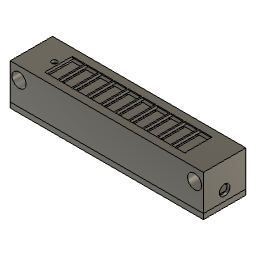
USB Power Distribution (Autodesk Fusion 360 design; units mm, degrees)
Autodesk Fusion 360 part; units mm, degrees
note: some values were not read from the file. Set by a fixed rule: which sketch regions a step uses.
sketch "Sketch1" plane through (0, 0, 0) normal (0, 0, 1) x (1, 0, 0) in component "USB PCB"
  line L0 (2, 0) -> (87.5, 0)
  line L1 (89.5, 2) -> (89.5, 16)
  line L2 (87.5, 18) -> (2, 18)
  line L3 (0, 16) -> (0, 2)
  circle A0 centre (2.7, 2.5) radius 1.75
  circle A1 centre (2.5, 15.5) radius 1.75
  circle A2 centre (87, 2.5) radius 1.75
  circle A3 centre (87, 15.5) radius 1.75
  arc A4 (2, 18) -> (0, 16) centre (2, 16) ccw
  arc A5 (89.5, 16) -> (87.5, 18) centre (87.5, 16) ccw
  arc A6 (87.5, 0) -> (89.5, 2) centre (87.5, 2) ccw
  arc A7 (0, 2) -> (2, 0) centre (2, 2) ccw
  line L4 (12.6, 1.25) -> (5.4, 1.25)
  line L5 (5.4, 1.25) -> (5.4, 16.75)
  line L6 (5.4, 16.75) -> (12.6, 16.75)
  line L7 (12.6, 16.75) -> (12.6, 1.25)
  line L8 (12.6, 1.25) -> (5.4, 16.75) construction
  line L9 (5.4, 1.25) -> (12.6, 16.75) construction
  line L10 (13.4, 16.75) -> (20.6, 16.75)
  line L11 (13.4, 1.25) -> (13.4, 16.75)
  line L12 (20.6, 16.75) -> (20.6, 1.25)
  line L13 (20.6, 1.25) -> (13.4, 1.25)
  line L14 (21.4, 16.75) -> (28.6, 16.75)
  line L15 (21.4, 1.25) -> (21.4, 16.75)
  line L16 (28.6, 16.75) -> (28.6, 1.25)
  line L17 (28.6, 1.25) -> (21.4, 1.25)
  line L18 (29.4, 16.75) -> (36.6, 16.75)
  line L19 (29.4, 1.25) -> (29.4, 16.75)
  line L20 (36.6, 16.75) -> (36.6, 1.25)
  line L21 (36.6, 1.25) -> (29.4, 1.25)
  line L22 (37.4, 16.75) -> (44.6, 16.75)
  line L23 (37.4, 1.25) -> (37.4, 16.75)
  line L24 (44.6, 16.75) -> (44.6, 1.25)
  line L25 (44.6, 1.25) -> (37.4, 1.25)
  line L26 (45.4, 16.75) -> (52.6, 16.75)
  line L27 (45.4, 1.25) -> (45.4, 16.75)
  line L28 (52.6, 16.75) -> (52.6, 1.25)
  line L29 (52.6, 1.25) -> (45.4, 1.25)
  line L30 (53.4, 16.75) -> (60.6, 16.75)
  line L31 (53.4, 1.25) -> (53.4, 16.75)
  line L32 (60.6, 16.75) -> (60.6, 1.25)
  line L33 (60.6, 1.25) -> (53.4, 1.25)
  line L34 (61.4, 16.75) -> (68.6, 16.75)
  line L35 (61.4, 1.25) -> (61.4, 16.75)
  line L36 (68.6, 16.75) -> (68.6, 1.25)
  line L37 (68.6, 1.25) -> (61.4, 1.25)
  line L38 (69.4, 16.75) -> (76.6, 16.75)
  line L39 (69.4, 1.25) -> (69.4, 16.75)
  line L40 (76.6, 16.75) -> (76.6, 1.25)
  line L41 (76.6, 1.25) -> (69.4, 1.25)
  line L42 (77.4, 16.75) -> (84.6, 16.75)
  line L43 (77.4, 1.25) -> (77.4, 16.75)
  line L44 (84.6, 16.75) -> (84.6, 1.25)
  line L45 (84.6, 1.25) -> (77.4, 1.25)
  circle A8 centre (3, 9) radius 2
  point P0 (89.5, 18)
  point P1 (0, 18)
  point P2 (9, 9)
  dimension "d1" = 18
  dimension "d2" = 89.5
  dimension "d3" = 3.5
  dimension "d4" = 2.7
  dimension "d5" = 3.5
  dimension "d6" = 2.5
  dimension "d7" = 3.5
  dimension "d8" = 3.5
  dimension "d9" = 15.5
  dimension "d10" = 2.5
  dimension "d11" = 87
  dimension "d12" = 2.5
  dimension "d13" = 87
  dimension "d14" = 15.5
  dimension "d15" = 2
  dimension "d16" = 2
  dimension "d17" = 9
  dimension "d18" = 15.5
  dimension "d19" = 9
  dimension "d20" = 7.2
  dimension "d23" = 8
  dimension "d24" = 0
  dimension "d29" = 4
  dimension "d30" = 3
  constraint horizontal L0
  constraint vertical L1
  constraint horizontal L2
  constraint vertical L3
  constraint coincident P1 L2
  constraint coincident P1 L3
  constraint tangent L2 A4
  constraint tangent L3 A4
  constraint coincident P0 L1
  constraint coincident P0 L2
  constraint tangent L1 A5
  constraint tangent L2 A5
  constraint tangent L0 A6
  constraint tangent L1 A6
  constraint equal A5 A6
  constraint coincident origin L0
  constraint coincident origin L3
  constraint tangent L0 A7
  constraint tangent L3 A7
  constraint equal A5 A7
  constraint perpendicular L4 L5
  constraint parallel L4 L6
  constraint parallel L5 L7
  constraint horizontal L4
  constraint coincident L8 P2
  constraint coincident L9 P2
  measures "d1" distance of origin P1
  measures "d2" distance of P0 P1
  measures "d3" diameter of A0
  measures "d4" distance of L3 A0.centre
  measures "d5" diameter of A1
  measures "d6" distance of L3 A1.centre
  measures "d7" diameter of A2
  measures "d8" diameter of A3
  measures "d9" distance of L0 A1.centre
  measures "d10" distance of L0 A0.centre
  measures "d11" distance of L3 A2.centre
  measures "d12" distance of L0 A2.centre
  measures "d13" distance of L3 A3.centre
  measures "d14" distance of L0 A3.centre
  measures "d15" radius of A4
  measures "d16" radius of A5
  measures "d17" distance of L3 P2
  measures "d18" distance of L4.start L6.end
  measures "d19" distance of L0 P2
  measures "d20" distance of L5 L7
  measures "d29" diameter of A8
  measures "d30" distance of L3 A8.centre
extrude "Extrude3" add sketch "Sketch1" along normal blind 7.5 contours A8 makes body 1 in component "USB PCB"
extrude "Extrude1" add sketch "Sketch1" against normal blind 1.6 separate body contours L0 L1 L2 L3 A4 A5 A6 A7 | L4 L5 L6 L7 | L10 L11 L12 L13 | L14 L15 L16 L17 | L18 L19 L20 L21 | L22 L23 L24 L25 | L26 L27 L28 L29 | L30 L31 L32 L33 | L34 L35 L36 L37 | L38 L39 L40 L41 | L42 L43 L44 L45 | A8 makes body 2 in component "USB PCB"
extrude "Extrude2" add sketch "Sketch1" along normal blind 13 contours L4 L5 L6 L7 | L10 L11 L12 L13 | L14 L15 L16 L17 | L18 L19 L20 L21 | L22 L23 L24 L25 | L26 L27 L28 L29 | L30 L31 L32 L33 | L34 L35 L36 L37 | L38 L39 L40 L41 | L42 L43 L44 L45 bodies 2 in component "USB PCB"
fillet "Fillet1" radius 2 1 edges at (1.1353, 8.2768, 7.5) on bodies 1 in component "USB PCB"
sketch "Sketch1 (2)" plane through (0, 0, 0) normal (0, 0, 1) x (1, 0, 0) in component "Bottom"
  line L0 (-10, 21) -> (99.5, 21)
  line L1 (99.5, 21) -> (99.5, -3)
  line L2 (99.5, -3) -> (-10, -3)
  line L3 (-10, -3) -> (-10, 21)
  line L4 (0, 16) -> (0, 2)
  line L5 (89.5, 2) -> (89.5, 16)
  circle A0 centre (87, 15.5) radius 3.25
  circle A1 centre (87, 2.5) radius 3.25
  circle A2 centre (2.5, 15.5) radius 3.25
  circle A3 centre (2.7, 2.5) radius 3.25
  line L6 (97.7, 19.2) -> (97.7, -1.2)
  line L7 (97.7, -1.2) -> (-8.2, -1.2)
  line L8 (-8.2, -1.2) -> (-8.2, 19.2)
  line L9 (-8.2, 19.2) -> (97.7, 19.2)
  line L10 (96.1, 0.4) -> (-6.6, 0.4)
  line L11 (-6.6, 0.4) -> (-6.6, 17.6)
  line L12 (-6.6, 17.6) -> (96.1, 17.6)
  line L13 (96.1, 17.6) -> (96.1, 0.4)
  line L14 (87, -1.2) -> (87, 19.2)
  line L15 (2.5, 19.2) -> (2.5, -1.2)
  circle A4 centre (2.5, 15.5) radius 1.6
  circle A5 centre (2.7, 2.5) radius 1.6
  circle A6 centre (87, 15.5) radius 1.6
  circle A7 centre (87, 2.5) radius 1.6
  circle A8 centre (92.983, 9) radius 3
  point P0 (2.5, 15.5)
  point P1 (2.7, 2.5)
  point P2 (87, 2.5)
  point P3 (87, 15.5)
  dimension "d34" = 10
  dimension "d35" = 10
  dimension "d38" = 6.5
  dimension "d39" = 6.5
  dimension "d40" = 6.5
  dimension "d41" = 6.5
  dimension "d42" = 1.8
  dimension "d43" = 1.8
  dimension "d44" = 1.8
  dimension "d45" = 1.8
  dimension "d46" = 1.6
  dimension "d47" = 3.2
  dimension "d48" = 3.2
  dimension "d49" = 3.2
  dimension "d50" = 3.2
  dimension "d93" = 6
  constraint horizontal L0
  constraint vertical L1
  constraint horizontal L2
  constraint vertical L3
  constraint coincident P3 A0.centre
  constraint coincident P2 A1.centre
  constraint coincident P0 A2.centre
  constraint coincident P1 A3.centre
  constraint parallel L1 L6
  constraint perpendicular L1 L7
  constraint perpendicular L7 L8
  constraint perpendicular L6 L9
  constraint coincident L7 L14.start
  constraint coincident L9 L14.end
  constraint perpendicular L9 L14
  constraint coincident L9 L15.start
  constraint coincident L7 L15.end
  constraint perpendicular L7 L15
  constraint concentric A2 A4
  constraint concentric A3 A5
  constraint concentric A1 A7
  measures "d34" distance of L3 L4
  measures "d35" distance of L1 L5
  measures "d38" diameter of A0
  measures "d39" diameter of A1
  measures "d40" diameter of A2
  measures "d41" diameter of A3
  measures "d42" distance of L0 L9
  measures "d43" distance of L1 L6
  measures "d44" distance of L2 L7
  measures "d45" distance of L3 L8
  measures "d47" diameter of A4
  measures "d48" diameter of A5
  measures "d49" diameter of A6
  measures "d50" diameter of A7
  measures "d93" diameter of A8
extrude "Extrude1'" add sketch "Sketch1 (2)" along normal blind 1.5 separate body contours A2 A3 L7 L8 L9 L10 L11 L12 L15 | A0 A1 L6 L7 L9 L10 L12 L13 L14 makes body 3 at (-7.6667, 6.1333, 0) makes body 4 at (97.1667, 6.1333, 0) in component "Bottom"
extrude "Extrude2'" add sketch "Sketch1 (2)" along normal blind 1.9 contours A2 L12 L15 A4 | A3 L10 L15 A5 | A2 L12 L15 | A2 L12 L15 A4 | A3 L10 L15 A5 | A3 L10 L15 | A2 L12 L15 | A3 L10 L15 | A0 L12 L14 A6 | A0 L12 L14 | A1 L10 L14 | A1 L10 L14 A7 | A0 L12 L14 | A0 L12 L14 A6 | A1 L10 L14 A7 | A1 L10 L14 bodies 3 4 in component "Bottom"
extrude "Extrude3'" add sketch "Sketch1 (2)" against normal blind 3 contours L0 L1 L2 L3 | L4 A2 A3 L15 | L4 A2 A3 L10 L11 L12 | A2 L12 L15 A4 | A3 L10 L15 A5 | A2 A3 L7 L8 L9 L10 L11 L12 L15 | A2 L12 L15 | A2 L12 L15 A4 | A0 A1 A2 A3 L10 L12 L14 L15 | A3 L10 L15 A5 | A3 L10 L15 | A0 A2 L9 L12 L14 L15 | A2 L12 L15 | A3 L10 L15 | A1 A3 L7 L10 L14 L15 | A0 L12 L14 A6 | A0 L12 L14 | A0 A1 L6 L7 L9 L10 L12 L13 L14 | A1 L10 L14 | A1 L10 L14 A7 | A0 L12 L14 | A0 L12 L14 A6 | L5 A0 A1 L14 | A1 L10 L14 A7 | A1 L10 L14 | L5 A0 A1 L10 L12 L13 | A8 bodies 3 4 in component "Bottom"
extrude "Extrude4" cut sketch "Sketch1 (2)" against normal blind 2 from surface at -1 contours A2 L12 L15 A4 | A3 L10 L15 A5 | A2 L12 L15 | A2 L12 L15 A4 | A3 L10 L15 A5 | A3 L10 L15 | A2 L12 L15 | A3 L10 L15 | A0 L12 L14 A6 | A0 L12 L14 | A1 L10 L14 | A1 L10 L14 A7 | A0 L12 L14 | A0 L12 L14 A6 | A1 L10 L14 A7 | A1 L10 L14 bodies 3 in component "Bottom"
sketch "Sketch1 (3)" plane through (0, 0, 0) normal (0, 0, 1) x (1, 0, 0) in component "Top"
  line L0 (-10, 21) -> (99.5, 21)
  line L1 (-10, -3) -> (-10, 21)
  line L2 (99.5, -3) -> (-10, -3)
  line L3 (99.5, 21) -> (99.5, -3)
  circle A0 centre (2.5, 15.5) radius 1.1
  circle A1 centre (2.7, 2.5) radius 1.1
  circle A2 centre (87, 15.5) radius 1.1
  circle A3 centre (87, 2.5) radius 1.1
  line L4 (97.9, -1.4) -> (-8.4, -1.4)
  line L5 (-8.4, -1.4) -> (-8.4, 19.4)
  line L6 (-8.4, 19.4) -> (97.9, 19.4)
  line L7 (97.9, 19.4) -> (97.9, -1.4)
  point P0 (2.5, 15.5)
  point P1 (2.7, 2.5)
  point P2 (87, 15.5)
  point P3 (87, 2.5)
  dimension "d60" = 2.2
  dimension "d61" = 2.2
  dimension "d62" = 2.2
  dimension "d63" = 2.2
  dimension "d64" = 1.6
  constraint coincident P0 A0.centre
  constraint coincident P1 A1.centre
  constraint coincident P2 A2.centre
  constraint coincident P3 A3.centre
  measures "d60" diameter of A0
  measures "d61" diameter of A1
  measures "d62" diameter of A2
  measures "d63" diameter of A3
extrude "Extrude1''" add sketch "Sketch1 (3)" along normal blind 20 separate body contours L0 L1 L2 L3 makes body 5 in component "Top"
extrude "Extrude2''" add sketch "Sketch1 (3)" along normal blind 1.6 from surface at 18.6 contours L0 L1 L2 L3 | A0 | A1 | A2 | A3 | L4 L5 L6 L7 bodies 5 in component "Top"
sketch "Sketch2" plane through (0, 0, 20.2) normal (0, 0, 1) x (-1, 0, 0) in component "Top"
  line L0 (-5.4, -1.25) -> (-5.4, -16.75)
  line L1 (-12.6, -16.75) -> (-5.4, -16.75)
  line L2 (-5.4, -16.75) -> (-5.4, -1.25)
  line L3 (-5.4, -1.25) -> (-12.6, -1.25)
  line L4 (-12.6, -1.25) -> (-12.6, -16.75)
  line L5 (-20.6, -1.25) -> (-20.6, -16.75)
  line L6 (-20.6, -16.75) -> (-13.4, -16.75)
  line L7 (-13.4, -16.75) -> (-13.4, -1.25)
  line L8 (-13.4, -1.25) -> (-20.6, -1.25)
  line L9 (-28.6, -1.25) -> (-28.6, -16.75)
  line L10 (-28.6, -16.75) -> (-21.4, -16.75)
  line L11 (-21.4, -16.75) -> (-21.4, -1.25)
  line L12 (-21.4, -1.25) -> (-28.6, -1.25)
  line L13 (-36.6, -1.25) -> (-36.6, -16.75)
  line L14 (-36.6, -16.75) -> (-29.4, -16.75)
  line L15 (-29.4, -16.75) -> (-29.4, -1.25)
  line L16 (-29.4, -1.25) -> (-36.6, -1.25)
  line L17 (-44.6, -1.25) -> (-44.6, -16.75)
  line L18 (-44.6, -16.75) -> (-37.4, -16.75)
  line L19 (-37.4, -16.75) -> (-37.4, -1.25)
  line L20 (-37.4, -1.25) -> (-44.6, -1.25)
  line L21 (-52.6, -1.25) -> (-52.6, -16.75)
  line L22 (-52.6, -16.75) -> (-45.4, -16.75)
  line L23 (-45.4, -16.75) -> (-45.4, -1.25)
  line L24 (-45.4, -1.25) -> (-52.6, -1.25)
  line L25 (-60.6, -1.25) -> (-60.6, -16.75)
  line L26 (-60.6, -16.75) -> (-53.4, -16.75)
  line L27 (-53.4, -16.75) -> (-53.4, -1.25)
  line L28 (-53.4, -1.25) -> (-60.6, -1.25)
  line L29 (-68.6, -1.25) -> (-68.6, -16.75)
  line L30 (-68.6, -16.75) -> (-61.4, -16.75)
  line L31 (-61.4, -16.75) -> (-61.4, -1.25)
  line L32 (-61.4, -1.25) -> (-68.6, -1.25)
  line L33 (-76.6, -1.25) -> (-76.6, -16.75)
  line L34 (-76.6, -16.75) -> (-69.4, -16.75)
  line L35 (-69.4, -16.75) -> (-69.4, -1.25)
  line L36 (-69.4, -1.25) -> (-76.6, -1.25)
  line L37 (-84.6, -1.25) -> (-84.6, -16.75)
  line L38 (-84.6, -16.75) -> (-77.4, -16.75)
  line L39 (-77.4, -16.75) -> (-77.4, -1.25)
  line L40 (-77.4, -1.25) -> (-84.6, -1.25)
  circle A0 centre (-3, -9) radius 1.5
  circle A1 centre (-2.5, -15.5) radius 2.5
  circle A2 centre (-2.7, -2.5) radius 2.5
  circle A3 centre (-87, -15.5) radius 2.5
  circle A4 centre (-87, -2.5) radius 2.5
  circle A5 centre (-2.5, -15.5) radius 1.25
  circle A6 centre (-2.7, -2.5) radius 1.25
  circle A7 centre (-87, -2.5) radius 1.25
  circle A8 centre (-87, -15.5) radius 1.25
  line L41 (-99.5, -21) -> (10, -21)
  line L42 (10, -21) -> (10, 3)
  line L43 (10, 3) -> (-99.5, 3)
  line L44 (-99.5, 3) -> (-99.5, -21)
  point P0 (-3, -9)
  point P1 (-2.5, -15.5)
  point P2 (-2.7, -2.5)
  point P3 (-87, -15.5)
  point P4 (-87, -2.5)
  dimension "d70" = 3
  dimension "d97" = 5
  dimension "d98" = 5
  dimension "d99" = 5
  dimension "d100" = 5
  dimension "d101" = 2.5
  dimension "d102" = 2.5
  dimension "d103" = 2.5
  dimension "d104" = 2.5
  constraint coincident P0 A0.centre
  constraint coincident P1 A1.centre
  constraint coincident P2 A2.centre
  constraint coincident P3 A3.centre
  constraint coincident P4 A4.centre
  constraint concentric A1 A5
  constraint concentric A4 A7
  measures "d70" diameter of A0
  measures "d97" diameter of A1
  measures "d98" diameter of A2
  measures "d99" diameter of A3
  measures "d100" diameter of A4
  measures "d101" diameter of A5
  measures "d102" diameter of A6
  measures "d103" diameter of A7
  measures "d104" diameter of A8
extrude "Extrude3''" cut sketch "Sketch2" against normal blind 1.6 contours L0 L1 L2 L3 L4 | L5 L6 L7 L8 | L9 L10 L11 L12 | L13 L14 L15 L16 | L17 L18 L19 L20 | L21 L22 L23 L24 | L25 L26 L27 L28 | L29 L30 L31 L32 | L33 L34 L35 L36 | L37 L38 L39 L40 A3 A4 | L37 A4 | L37 A3 | A0 picked at (-84.5815, -2.3433) picked at (-84.5815, -15.3433) bodies 5 in component "Top"
sketch "Sketch3" plane through (0, -3, 0) normal (0, -1, 0) x (1, 0, 0) in component "Top"
  line L0 (-10, 20.2) -> (-10, 0)
  line L1 (-10, 0) -> (99.5, 0)
  line L2 (99.5, 0) -> (99.5, 20.2)
  circle A0 centre (-5, 13.2) radius 5
  circle A1 centre (-5, 13.2) radius 2
  circle A2 centre (94.5, 13.2) radius 2
  circle A3 centre (94.5, 13.2) radius 5
  circle A4 centre (-5, 13.2) radius 4
  circle A5 centre (94.5, 13.2) radius 4
  line L3 (99.5, 20.2) -> (-10, 20.2)
  dimension "d73" = 10
  dimension "d74" = 4
  dimension "d75" = 4
  dimension "d76" = 10
  dimension "d77" = 5
  dimension "d78" = 5
  dimension "d83" = 8
  dimension "d84" = 8
  dimension "d107" = 7
  dimension "d108" = 7
  constraint concentric A0 A1
  constraint concentric A2 A3
  constraint concentric A1 A4
  constraint concentric A2 A5
  measures "d73" diameter of A0
  measures "d74" diameter of A1
  measures "d75" diameter of A2
  measures "d76" diameter of A3
  measures "d77" distance of L0 A0.centre
  measures "d78" distance of L2 A2.centre
  measures "d83" diameter of A4
  measures "d84" diameter of A5
  measures "d107" distance of A0.centre L3
  measures "d108" distance of A2.centre L3
extrude "Extrude4'" add sketch "Sketch3" against normal up to surface (22.4 mm away) contours A0 | A3 | A4 | A5 bodies 5 in component "Top"
extrude "Extrude5" cut sketch "Sketch3" against normal up to surface (24 mm away) contours A1 | A2 bodies 5 in component "Top"
extrude "Extrude6" cut sketch "Sketch3" against normal up to surface (21 mm away) contours A4 | A5 bodies 5 in component "Top"
chamfer "Chamfer1" distance 1.5 angle 45 2 edges at (-6.8647, 18, 12.4768) (92.6353, 18, 12.4768) on bodies 5 in component "Top"
sketch "Sketch4" plane through (99.5, 0, 0) normal (1, 0, 0) x (0, 1, 0) in component "Top"
  line L0 (-3, 20.2) -> (-3, 0)
  line L1 (-3, 0) -> (21, 0)
  line L2 (21, 0) -> (21, 20.2)
  circle A0 centre (9, 5.5) radius 3
  line L3 (21, 20.2) -> (-3, 20.2)
  dimension "d90" = 6
  measures "d90" diameter of A0
extrude "Extrude7" cut sketch "Sketch4" against normal up to surface (1.6 mm away) contours A0 bodies 5 in component "Top"
extrude "Extrude5'" cut sketch "Sketch1 (2)" against normal up to surface (3 mm away) contours A8 bodies 3 in component "Bottom"
chamfer "Chamfer2" distance 1 angle 45 20 edges at (9, 16.75, 18.6) (17, 16.75, 18.6) (25, 16.75, 18.6) (33, 16.75, 18.6) (41, 16.75, 18.6) (49, 16.75, 18.6) (57, 16.75, 18.6) (65, 16.75, 18.6) (73, 16.75, 18.6) (81, 16.75, 18.6) (9, 1.25, 18.6) (17, 1.25, 18.6) (25, 1.25, 18.6) (33, 1.25, 18.6) (41, 1.25, 18.6) (49, 1.25, 18.6) (57, 1.25, 18.6) (65, 1.25, 18.6) (73, 1.25, 18.6) (81, 1.25, 18.6) on bodies 5 in component "Top"
extrude "Extrude8" add sketch "Sketch2" against normal blind 14 contours L37 A4 | L37 A3 | A1 | A2 picked at (-84.9833, -2.5) picked at (-84.9833, -15.5) bodies 5 in component "Top"
component "USB PCB" placed x (1, 0, 0) y (0, 1, 0) z (0, 0, 1) at (0, 0, 4.6)
component "Bottom" placed x (1, 0, 0) y (0, 1, 0) z (0, 0, 1) at (0, 0, 0)
component "Top" placed x (1, 0, 0) y (0, 1, 0) z (0, 0, 1) at (0, 0, 0)
equation "d53 = 3.5 mm - 1.6 mm"
